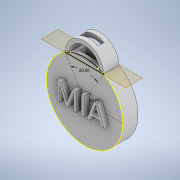
# Autodesk Inventor part: MIA Pendant 2
Saved by Autodesk Inventor 2020 (Build 240168000, 168)
## iProperties
Created: 2019-10-01
Part Number: MIA Pendant 2
Material: Generic
Document SubType Name: Modeling
Designer: Alex
Density: 1 g/cm^3
Appearance: Default
Author: Alex
Autodesk Inventor part; units mm, degrees
ref_plane "YZ Plane" through (0, 0, 0) normal (1, 0, 0) x (0, 1, 0)
ref_plane "XZ Plane" through (0, 0, 0) normal (0, 1, 0) x (-1, 0, 0)
ref_plane "XY Plane" through (0, 0, 0) normal (0, 0, 1) x (1, 0, 0)
sketch "Sketch1" plane through (0, 0, 0) normal (0, 0, 1) x (1, 0, 0)
  circle A0 centre (0, 0) radius 12.7
  arc A1 (3.287, 12.2673) -> (-3.287, 12.2673) centre (0, 0) ccw
  line L0 (0, 0) -> (3.287, 12.2673) construction
  line L1 (0, 0) -> (12.7, 0) construction
  line L2 (0, 0) -> (-3.287, 12.2673) construction
  line L3 (-3.287, 12.2673) -> (3.287, 12.2673)
  point P0 (3.287, 12.2673)
  point P1 (-3.287, 12.2673)
  dimension "d0" = 25.4
  dimension "d1" = 12.7
  dimension "d2" = 75
  dimension "d3" = 30
  constraints: 8 end point, 2 centre point, 2 coincident, 2 point on circle, 1 equal length, 1 horizontal
  measures "d0" diameter of A0
  measures "d1" radius of A1
  measures "d2" angle of L1 L0
  measures "d3" angle of L0 L2
extrude "Extrusion1" add sketch "Sketch1" along normal blind 5.08 contours A0 L3 picked at (4.079, -0.9801)
sketch "Sketch3" plane through (0, 0, 5.08) normal (0, 0, 1) x (1, 0, 0)
  arc A0 (-3.287, 12.2673) -> (3.287, 12.2673) centre (0, 0) ccw projected
  arc A1 (6.35, 10.9985) -> (-6.35, 10.9985) centre (0, 0) ccw
  line L0 (0, 0) -> (6.35, 10.9985) construction
  line L1 (0, 0) -> (12.7, 0) construction
  line L2 (0, 0) -> (-6.35, 10.9985) construction
  line L3 (-6.35, 10.9985) -> (6.35, 10.9985)
  dimension "d12" = 60
  dimension "d13" = 60
  constraints: 8 end point, 3 point on circle, 1 centre point, 1 coincident, 1 equal length, 1 horizontal
  measures "d12" angle of L1 L0
  measures "d13" angle of L0 L2
ref_plane "Work Plane1" through (-6.35, 10.9985, 5.08) normal (0, 1, 0) x (1, 0, 0)
sketch "Sketch4" plane through (-6.35, 10.9985, 5.08) normal (0, 1, 0) x (1, 0, 0)
  line L0 (-6.35, 0) -> (19.05, 0) projected
  line L1 (-6.35, 5.08) -> (19.05, 5.08) projected
  line L2 (-0.0044, 0) -> (12.6956, 0)
  line L3 (12.6956, 0) -> (12.6956, 5.08)
  line L4 (12.6956, 5.08) -> (-0.0044, 5.08)
  line L5 (-0.0044, 5.08) -> (-0.0044, 0)
  line L6 (-0.0044, 5.08) -> (1.2656, 5.08)
  line L7 (1.2656, 5.08) -> (1.2656, 0)
  line L8 (1.2656, 0) -> (-0.0044, 0)
  line L9 (-0.0044, 0) -> (-0.0044, 5.08)
  line L10 (12.6956, 0) -> (11.4256, 0)
  line L11 (11.4256, 0) -> (11.4256, 5.08)
  line L12 (11.4256, 5.08) -> (12.6956, 5.08)
  line L13 (12.6956, 5.08) -> (12.6956, 0)
  line L14 (6.35, 5.08) -> (6.3456, 0)
  point P0 (3.063, 0)
  point P1 (9.637, 0)
  point P2 (3.063, 5.08)
  point P3 (9.637, 5.08)
  dimension "d15" = 12.7
  dimension "d16" = 1.27
  dimension "d17" = 1.27
  constraints: 26 end point, 6 parallel, 4 point on line, 3 horizontal, 3 perpendicular, 1 midpoint
  measures "d15" distance of L4.end L3.end
  measures "d16" distance of L7.end L8.end
  measures "d17" distance of L11.end L12.end
revolve "Revolution1" add sketch "Sketch4" angle 180 about axis through (0, 10.9985, 0) along (-0.0009, 0, 1) contours L11 L1 L3 L0
sketch "Sketch5" plane through (0, 0, 5.08) normal (0, 0, 1) x (1, 0, 0)
  line L0 (6.35, -3.175) -> (-6.35, -3.175)
  line L1 (-6.35, -3.175) -> (-6.35, 3.175)
  line L2 (-6.35, 3.175) -> (6.35, 3.175)
  line L3 (6.35, 3.175) -> (6.35, -3.175)
  line L4 (6.35, -3.175) -> (-6.35, 3.175) construction
  line L5 (-6.35, -3.175) -> (6.35, 3.175) construction
  line L6 (-9.525, 3.175) -> (9.525, 3.175) construction
  line L7 (9.525, 3.175) -> (9.525, -3.0049) construction
  line L8 (9.525, -3.0049) -> (-9.525, -3.0049) construction
  line L9 (-9.525, -3.0049) -> (-9.525, 3.175) construction
  line L10 (-6.35, 3.175) -> (-9.525, 3.175)
  line L11 (-0.9161, -2.921) -> (-1.917, -2.921)
  line L12 (-1.917, -2.921) -> (-1.917, 1.0261)
  spline S0 degree 2 poles (-1.917, 1.0261) (-1.917, 1.5125) (-1.8605, 2.2137) knots 0 0 0 1 1 1
  line L13 (-1.8605, 2.2137) -> (-1.8774, 2.2137)
  spline S1 degree 2 poles (-1.8774, 2.2137) (-1.9679, 1.8122) (-2.0414, 1.6369) knots 0 0 0 1 1 1
  line L14 (-2.0414, 1.6369) -> (-3.8623, -2.921)
  line L15 (-3.8623, -2.921) -> (-4.5579, -2.921)
  line L16 (-4.5579, -2.921) -> (-6.3844, 1.6029)
  spline S2 degree 2 poles (-6.3844, 1.6029) (-6.4579, 1.8009) (-6.5427, 2.2137) knots 0 0 0 1 1 1
  line L17 (-6.5427, 2.2137) -> (-6.5597, 2.2137)
  spline S3 degree 2 poles (-6.5597, 2.2137) (-6.5258, 1.8461) (-6.5258, 1.0148) knots 0 0 0 1 1 1
  line L18 (-6.5258, 1.0148) -> (-6.5258, -2.921)
  line L19 (-6.5258, -2.921) -> (-7.4645, -2.921)
  line L20 (-7.4645, -2.921) -> (-7.4645, 3.175)
  line L21 (-7.4645, 3.175) -> (-6.0395, 3.175)
  line L22 (-6.0395, 3.175) -> (-4.4391, -0.8852)
  spline S4 degree 2 poles (-4.4391, -0.8852) (-4.2525, -1.3546) (-4.1959, -1.5808) knots 0 0 0 1 1 1
  line L23 (-4.1959, -1.5808) -> (-4.179, -1.5808)
  spline S5 degree 2 poles (-4.179, -1.5808) (-4.0206, -1.1001) (-3.9245, -0.8683) knots 0 0 0 1 1 1
  line L24 (-3.9245, -0.8683) -> (-2.2902, 3.175)
  line L25 (-2.2902, 3.175) -> (-0.9161, 3.175)
  line L26 (-0.9161, 3.175) -> (-0.9161, -2.921)
  line L27 (1.623, -2.921) -> (0.5768, -2.921)
  line L28 (0.5768, -2.921) -> (0.5768, 3.175)
  line L29 (0.5768, 3.175) -> (1.623, 3.175)
  line L30 (1.623, 3.175) -> (1.623, -2.921)
  line L31 (8.1318, -2.921) -> (7.0234, -2.921)
  line L32 (7.0234, -2.921) -> (6.4749, -1.3716)
  line L33 (6.4749, -1.3716) -> (4.0772, -1.3716)
  line L34 (4.0772, -1.3716) -> (3.5456, -2.921)
  line L35 (3.5456, -2.921) -> (2.4429, -2.921)
  line L36 (2.4429, -2.921) -> (4.7275, 3.175)
  line L37 (4.7275, 3.175) -> (5.8641, 3.175)
  line L38 (5.8641, 3.175) -> (8.1318, -2.921)
  line L39 (6.2034, -0.5459) -> (5.3609, 1.8857)
  spline S6 degree 2 poles (5.3609, 1.8857) (5.3213, 2.0101) (5.276, 2.2702) knots 0 0 0 1 1 1
  line L40 (5.276, 2.2702) -> (5.2591, 2.2702)
  spline S7 degree 2 poles (5.2591, 2.2702) (5.2251, 2.0271) (5.1742, 1.8857) knots 0 0 0 1 1 1
  line L41 (5.1742, 1.8857) -> (4.3373, -0.5459)
  line L42 (4.3373, -0.5459) -> (6.2034, -0.5459)
  point P0 (0, 0)
  dimension "d19" = 12.7
  dimension "d20" = 6.35
  dimension "d21" = 19.05
  dimension "d22" = 3.175
  constraints: 14 end point, 2 horizontal, 2 midpoint, 2 parallel, 1 perpendicular, 2 other
  measures "d19" distance of L0.start L0.end
  measures "d20" distance of L0.end L1.end
  measures "d21" distance of L6.start L6.end
  measures "d22" distance of L1.end L10.end
extrude "Extrusion3" add sketch "Sketch5" along normal blind 1.5875 contours L33 L34 L35 L36 L2 L38 L3 | L3 L38 L31 L32 L33 | L16 S2 L17 S3 L18 L19 L20 L10 L1 | L1 L2 L22 S4 L23 S5 L24 L26 L11 L12 S0 L13 S1 L14 L15 L16 | L30 L27 L28 L2
sketch "Sketch2" plane through (-3.287, 12.2673, 0) normal (0, 1, 0) x (1, 0, 0)
  line L0 (6.574, 0) -> (0, 0) projected
  line L1 (6.574, -5.08) -> (0, -5.08) projected
  line L2 (0, 0) -> (6.574, 0)
  line L3 (6.574, 0) -> (6.574, -5.08)
  line L4 (6.574, -5.08) -> (0, -5.08)
  line L5 (0, -5.08) -> (0, 0)
  line L6 (3.287, 0) -> (3.287, -5.08)
  line L7 (0.287, -1.54) -> (6.287, -1.54)
  line L8 (6.287, -1.54) -> (6.287, -3.54)
  line L9 (6.287, -3.54) -> (0.287, -3.54)
  line L10 (0.287, -3.54) -> (0.287, -1.54)
  line L11 (0.287, -1.54) -> (6.287, -3.54) construction
  line L12 (6.287, -1.54) -> (0.287, -3.54) construction
  point P0 (3.287, -2.54)
  dimension "d6" = 6.574
  dimension "d8" = 6
  dimension "d9" = 2
  constraints: 22 end point, 4 midpoint, 4 parallel, 3 perpendicular, 1 horizontal
  measures "d6" distance of L0.start L0.end
  measures "d8" distance of L7.start L7.end
  measures "d9" distance of L7.end L8.end
extrude "Extrusion2" cut sketch "Sketch2" along normal blind 12.7 and the other way blind 17 contours L7 L8 L9 L6 | L6 L9 L10 L7
body "Solid1"
